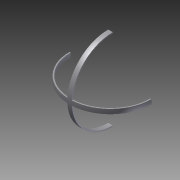
# Autodesk Inventor part: shell model
Saved by Autodesk Inventor 2012 (Build 160160000, 160)
## iProperties
Created: 2011-10-07
Part Number: shell model
Material: Default
Document SubType Name: Modeling
Designer: Antonella
Density: 1 g/cm^3
Author: Antonella
Autodesk Inventor part; units mm, degrees
ref_plane "YZ Plane" through (0, 0, 0) normal (1, 0, 0) x (0, 1, 0)
ref_plane "XZ Plane" through (0, 0, 0) normal (0, 1, 0) x (-1, 0, 0)
ref_plane "XY Plane" through (0, 0, 0) normal (0, 0, 1) x (1, 0, 0)
sketch "Sketch1" plane through (0, 0, 0) normal (0, 0, 1) x (1, 0, 0)
  line L0 (-137.16, 0) -> (22.86, 0) projected
  line L1 (0, -160.02) -> (0, 160.02) projected
  arc A0 (0, 114.3) -> (0, -114.3) centre (0, 0) ccw
  arc A1 (0, 111.125) -> (0, -111.125) centre (0, 0) ccw
  line L2 (0, 111.125) -> (0, 114.3)
  line L3 (0, -114.3) -> (0, -111.125)
  dimension "d6" = 3.175
  dimension "d7" = 228.6
  constraints: 4 end point, 4 point on circle, 3 point on line, 2 centre point, 2 collinear, 1 coincident
  measures "d6" radial gap between concentric circles of A0 A1
  measures "d7" distance of L2.end L3.start
revolve "Revolution1" add sketch "Sketch1" angle 180 about axis through (0, -10, 0) along (0, 1, 0) contours A0 L1 A1 L0 | L0 A1 L1 A0
sketch "Sketch2" plane through (0, 0, 0) normal (0, 0, -1) x (-1, 0, 0)
  circle A0 centre (0, 0) radius 114.3 projected
  line L0 (-6.35, 114.1235) -> (-6.35, 6.4165)
  line L1 (-6.35, 6.4165) -> (-114.1198, 6.4165)
  line L2 (160.02, 0) -> (-160.02, 0) projected
  line L3 (0, -160.02) -> (0, 160.02) projected
  line L4 (-114.3, 0.0665) -> (114.3, 0.0665) construction
  dimension "d2" = 6.35
  dimension "d3" = 6.35
  constraints: 6 end point, 4 point on circle, 2 perpendicular, 1 vertical
  measures "d2" distance between parallel lines of L0 L3
  measures "d3" distance between parallel lines of L4 L1
extrude "Extrusion1" cut sketch "Sketch2" against normal through all contours L0 L1 A0
mirror "Mirror1" about plane through (0, 0, 0) normal (0, 1, 0) of "Extrusion1"
mirror "Mirror2" about plane through (0, 0, 0) normal (1, 0, 0) of "Extrusion1", "Mirror1"
body "Solid1"
